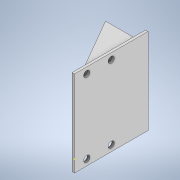
# Autodesk Inventor part: box3_camera_mount
Saved by Autodesk Inventor 2021.4 (Build 254397000, 397)
## iProperties
Created: 2023-09-26
Part Number: box3_camera_mount
Material: 一般
Document SubType Name: Modeling
Designer: ryusei
Density: 1 g/cm^3
Appearance: 既定
Author: ryusei
Autodesk Inventor part; units mm, degrees
ref_plane "YZ Plane" through (0, 0, 0) normal (1, 0, 0) x (0, 1, 0)
ref_plane "XZ Plane" through (0, 0, 0) normal (0, 1, 0) x (-1, 0, 0)
ref_plane "XY Plane" through (0, 0, 0) normal (0, 0, 1) x (1, 0, 0)
sketch "スケッチ3" plane through (0, 0, 0) normal (0, 1, 0) x (-1, 0, 0)
  line L0 (0, 0) -> (0, -60)
  line L1 (0, 0) -> (34.641, -60)
  line L2 (0, 0) -> (69.282, 0) construction
  line L3 (34.641, -60) -> (0, -60)
  dimension "d21" = 60
  dimension "d23" = 60
  constraints: 8 end point, 2 horizontal, 1 equal length, 1 vertical
  measures "d21" distance of L0.start L0.end
  measures "d23" angle of L1 L2
extrude "押し出し2" add sketch "スケッチ3" along normal blind 50
sketch "スケッチ4" plane through (0, 50, 0) normal (0, 1, 0) x (1, 0, 0)
  line L0 (0, 0) -> (0, 60) projected
  line L1 (0, 0) -> (0, 60)
  line L2 (0, 60) -> (-2, 60)
  line L3 (-2, 60) -> (-2, 0)
  line L4 (-2, 0) -> (0, 0)
  dimension "d26" = 2
  constraints: 8 end point, 3 equal length, 1 perpendicular
  measures "d26" distance of L2.end L0.end
extrude "押し出し3" add sketch "スケッチ4" along normal blind 10 and the other way blind 60
sketch "スケッチ5" plane through (-34.641, 0, -60) normal (-0.8660254, 0, 0.5) x (0.5, 0, 0.8660254)
  line L0 (65.282, 0) -> (65.282, 50) projected
  line L1 (0, 0) -> (65.282, 0) projected
  line L2 (0, 0) -> (0, 50) projected
  point P0 (69.282, 0)
  point P1 (10, 25)
  dimension "d32" = 25
  dimension "d68" = 10
  measures "d32" distance from line of L1 point (10, 25)
  measures "d68" distance from line of L2 point (10, 25)
hole "穴2" at (-29.641, 25, -51.3397) direction (0.8660254, 0, -0.5) diameter 11 end through all
sketch "スケッチ6" plane through (-34.641, 0, -60) normal (-0.8660254, 0, 0.5) x (0.5, 0, 0.8660254)
  point P0 (69.282, 0)
sketch "スケッチ12" plane through (-2, 50, -60) normal (-1, 0, 0) x (0, 0, 1)
  line L0 (60, -60) -> (60, 10) projected
  line L1 (60, -60) -> (0, -60) projected
  point P0 (60, -50)
  point P1 (50, -55)
  point P2 (30, -55)
  point P3 (50, 5)
  point P4 (30, 5)
  dimension "d51" = 10
  dimension "d52" = 5
  dimension "d55" = 20
  dimension "d58" = 60
  constraints: 1 horizontal, 1 vertical, 3 other
  measures "d51" distance from line of L0 point (50, -55)
  measures "d52" distance from line of L1 point (50, -55)
  measures "d55" distance of point (50, -55) point (30, -55)
  measures "d58" distance of point (50, -55) point (50, 5)
hole "穴4" at (-2, -5, -10) at (-2, -5, -30) at (-2, 55, -10) at (-2, 55, -30) direction (1, 0, 0) diameter 5.1 end through all
sketch "スケッチ13" plane through (-34.641, 0, -60) normal (-0.8660254, 0, 0.5) x (0.5, 0, 0.8660254)
  circle A0 centre (10, 25) radius 5.5
  line L0 (0, 0) -> (0, 50) projected
  line L1 (0, 0) -> (65.282, 0) projected
  point P0 (69.282, 0)
  dimension "d69" = 11
  dimension "d70" = 10
  dimension "d71" = 25
  constraints: 1 centre point
  measures "d69" diameter of A0
  measures "d70" distance from line of L0 A0.centre
  measures "d71" distance from line of L1 A0.centre
extrude "押し出し5" add sketch "スケッチ13" against normal blind 5
sketch "スケッチ14" plane through (-34.641, 0, -60) normal (-0.8660254, 0, 0.5) x (0.5, 0, 0.8660254)
  circle A0 centre (10, 25) radius 5.5 projected
  point P0 (69.282, 0)
  constraints: 1 coincident
hole "穴5" at (-29.641, 25, -51.3397) direction (0.8660254, 0, -0.5) diameter 6.3 end through all
